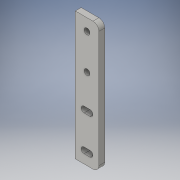
# Autodesk Inventor part: vrRig_v8_projMount02
Saved by Autodesk Inventor 2016 (Build 200138000, 138)
## iProperties
Created: 2018-01-13
Part Number: vrRig_v8_projMount02
Material: Generic
Document SubType Name: Modeling
Designer: harveylab
Density: 1 g/cm^3
Appearance: Default
Author: harveylab
Autodesk Inventor part; units mm, degrees
ref_plane "YZ Plane" through (0, 0, 0) normal (1, 0, 0) x (0, 1, 0)
ref_plane "XZ Plane" through (0, 0, 0) normal (0, 1, 0) x (-1, 0, 0)
ref_plane "XY Plane" through (0, 0, 0) normal (0, 0, 1) x (1, 0, 0)
sketch "Sketch1" plane through (0, 0, 0) normal (0, 0, 1) x (1, 0, 0)
  line L0 (19.05, 137.9474) -> (0, 137.9474)
  line L1 (0, 137.9474) -> (0, 0)
  line L2 (0, 0) -> (19.05, 0)
  arc A0 (19.05, 0) -> (25.4, 6.35) centre (19.05, 6.35) ccw
  line L3 (25.4, 6.35) -> (25.4, 131.5974)
  arc A1 (25.4, 131.5974) -> (19.05, 137.9474) centre (19.05, 131.5974) ccw
  circle A2 centre (12.7, 125.2474) radius 3.175
  circle A3 centre (12.7, 87.1474) radius 3.175
  arc A4 (9.525, 53.975) -> (9.525, 47.625) centre (9.525, 50.8) ccw
  arc A5 (15.875, 47.625) -> (15.875, 53.975) centre (15.875, 50.8) ccw
  line L4 (9.525, 53.975) -> (15.875, 53.975)
  line L5 (9.525, 47.625) -> (15.875, 47.625)
  arc A6 (9.525, 15.875) -> (9.525, 9.525) centre (9.525, 12.7) ccw
  arc A7 (15.875, 9.525) -> (15.875, 15.875) centre (15.875, 12.7) ccw
  line L6 (9.525, 15.875) -> (15.875, 15.875)
  line L7 (9.525, 9.525) -> (15.875, 9.525)
  point P0 (0, 0)
  constraints: 16 end point, 12 point on circle, 8 centre point
extrude "Extrusion1" add sketch "Sketch1" along normal blind 6.35
body "Solid1"
